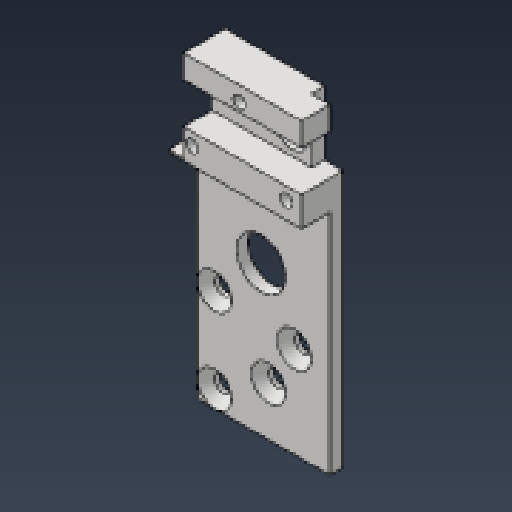
# Autodesk Inventor part: RightGearboxCover
Saved by Autodesk Inventor 2026.2 (Build 302298010, 298A)
## iProperties
Created: 2026-04-04
Part Number: RightGearboxCover
Material: Generic
Document SubType Name: Modeling
Designer: szymo
Density: 1 g/cm^3
Appearance: Default
Author: szymo
Autodesk Inventor part; units mm, degrees
ref_plane "YZ Plane" through (0, 0, 0) normal (1, 0, 0) x (0, 1, 0)
ref_plane "XZ Plane" through (0, 0, 0) normal (0, 1, 0) x (-1, 0, 0)
ref_plane "XY Plane" through (0, 0, 0) normal (0, 0, 1) x (1, 0, 0)
ref_plane "Work Plane1" through (0, -65.2958, -0.3) normal (0, 0, 1) x (1, 0, 0)
sketch "Sketch1" plane through (0, 0, 0) normal (0, 0, 1) x (1, 0, 0)
  circle A0 centre (13, -35.0012) radius 5
  circle A1 centre (13, -35.0012) radius 5.6
  circle A2 centre (8.3716, -9.3577) radius 1.0564
  circle A3 centre (20.6284, -19.6423) radius 1.0564 construction
  circle A4 centre (14.5, -14.5) radius 5 construction
  circle A5 centre (14.5, -14.5) radius 13.85 construction
  circle A6 centre (14.5, -14.5) radius 14.5 construction
  circle A7 centre (14.5, -55.2958) radius 14.5 construction
  circle A8 centre (14.5, -55.2958) radius 13.85 construction
  line L0 (27, 0) -> (0, 0)
  line L1 (0, 0) -> (0, -65.2958)
  line L2 (0, -65.2958) -> (27, -65.2958)
  line L3 (27, -65.2958) -> (27, 0)
  line L4 (1, -17) -> (1, -13.9)
  line L5 (1, -13.9) -> (0, -13.9)
  line L6 (0, -13.9) -> (0, -18)
  line L7 (0, -18) -> (2.4477, -18)
  arc A9 (2.5, -17.9298) -> (2.4477, -18) centre (9.2084, -22.9852) ccw
  line L8 (2.5, -17.9298) -> (2.5, -17)
  line L9 (2.5, -17) -> (1, -17)
  line L10 (3, 0) -> (3, -18.5)
  line L11 (3, -18.5) -> (0, -18.5)
  line L12 (3, -3) -> (27, -3)
  line L13 (27, -13) -> (3, -13)
  line L14 (23.2, 0) -> (23.2, -39.2749)
  arc A10 (9.6825, -42.5548) -> (9.605, -43.9808) centre (15.5954, -43.5915) ccw
  arc A11 (9.605, -43.9808) -> (10.0796, -44.1462) centre (13, -35.0012) ccw
  arc A12 (10.0796, -44.1462) -> (10.905, -42.9808) centre (5.6283, -40.1185) ccw
  arc A13 (10.905, -42.9808) -> (11.3255, -43.0795) centre (13, -35.0012) ccw
  arc A14 (11.3255, -43.0795) -> (11.5461, -44.4905) centre (17.3247, -42.8642) ccw
  arc A15 (11.5461, -44.4905) -> (12.0447, -44.5536) centre (13, -35.0012) ccw
  arc A16 (12.0447, -44.5536) -> (12.6098, -43.242) centre (6.8533, -41.5393) ccw
  arc A17 (12.6098, -43.242) -> (13.0416, -43.2511) centre (13, -35.0012) ccw
  arc A18 (13.0416, -43.2511) -> (13.5508, -44.5854) centre (18.865, -41.7932) ccw
  arc A19 (13.5508, -44.5854) -> (14.0517, -44.5434) centre (13, -35.0012) ccw
  arc A20 (14.0517, -44.5434) -> (14.3317, -43.143) centre (8.347, -42.6744) ccw
  arc A21 (14.3317, -43.143) -> (14.756, -43.0622) centre (13, -35.0012) ccw
  arc A22 (14.756, -43.0622) -> (15.5314, -44.2614) centre (20.1489, -40.4254) ccw
  arc A23 (15.5314, -44.2614) -> (16.0126, -44.1162) centre (13, -35.0012) ccw
  arc A24 (16.0126, -44.1162) -> (15.9954, -42.6882) centre (10.044, -43.4742) ccw
  arc A25 (15.9954, -42.6882) -> (16.3936, -42.5209) centre (13, -35.0012) ccw
  arc A26 (16.3936, -42.5209) -> (17.4014, -43.5327) centre (21.1205, -38.8205) ccw
  arc A27 (17.4014, -43.5327) -> (17.8419, -43.2907) centre (13, -35.0012) ccw
  arc A28 (17.8419, -43.2907) -> (17.5281, -41.8975) centre (11.8702, -43.9036) ccw
  arc A29 (17.5281, -41.8975) -> (17.8829, -41.651) centre (13, -35.0012) ccw
  arc A30 (17.8829, -41.651) -> (19.0791, -42.4312) centre (21.7371, -37.0487) ccw
  arc A31 (19.0791, -42.4312) -> (19.4596, -42.1029) centre (13, -35.0012) ccw
  arc A32 (19.4596, -42.1029) -> (18.863, -40.8053) centre (13.7458, -43.944) ccw
  arc A33 (18.863, -40.8053) -> (19.1587, -40.4905) centre (13, -35.0012) ccw
  arc A34 (19.1587, -40.4905) -> (20.491, -41.0049) centre (21.9719, -35.1874) ccw
  arc A35 (20.491, -41.0049) -> (20.795, -40.6047) centre (13, -35.0012) ccw
  arc A36 (20.795, -40.6047) -> (19.9416, -39.4595) centre (15.5888, -43.5935) ccw
  arc A37 (19.9416, -39.4595) -> (20.1654, -39.0901) centre (13, -35.0012) ccw
  arc A38 (20.1654, -39.0901) -> (21.5756, -39.3163) centre (21.8145, -33.318) ccw
  arc A39 (21.5756, -39.3163) -> (21.7896, -38.8615) centre (13, -35.0012) ccw
  arc A40 (21.7896, -38.8615) -> (20.7169, -37.9188) centre (17.3187, -42.8675) ccw
  arc A41 (20.7169, -37.9188) -> (20.859, -37.5109) centre (13, -35.0012) ccw
  arc A42 (20.859, -37.5109) -> (22.2853, -37.439) centre (21.272, -31.5221) ccw
  arc A43 (22.2853, -37.439) -> (22.4002, -36.9497) centre (13, -35.0012) ccw
  arc A44 (22.4002, -36.9497) -> (21.1548, -36.2506) centre (18.8598, -41.7976) ccw
  arc A45 (21.1548, -36.2506) -> (21.2091, -35.8221) centre (13, -35.0012) ccw
  arc A46 (21.2091, -35.8221) -> (22.5893, -35.4552) centre (20.3678, -29.8783) ccw
  arc A47 (22.5893, -35.4552) -> (22.5999, -34.9527) centre (13, -35.0012) ccw
  arc A48 (22.5999, -34.9527) -> (21.2364, -34.5278) centre (20.1448, -40.4308) ccw
  arc A49 (21.2364, -34.5278) -> (21.2003, -34.0974) centre (13, -35.0012) ccw
  arc A50 (21.2003, -34.0974) -> (22.4741, -33.4516) centre (19.1417, -28.4584) ccw
  arc A51 (22.4741, -33.4516) -> (22.38, -32.9579) centre (13, -35.0012) ccw
  arc A52 (22.38, -32.9579) -> (20.958, -32.8257) centre (21.1176, -38.8267) ccw
  arc A53 (20.958, -32.8257) -> (20.8332, -32.4122) centre (13, -35.0012) ccw
  arc A54 (20.8332, -32.4122) -> (21.9449, -31.5157) centre (17.6472, -27.3244) ccw
  arc A55 (21.9449, -31.5157) -> (21.7502, -31.0523) centre (13, -35.0012) ccw
  arc A56 (21.7502, -31.0523) -> (20.3318, -31.2187) centre (21.7355, -37.0553) ccw
  arc A57 (20.3318, -31.2187) -> (20.1238, -30.8402) centre (13, -35.0012) ccw
  arc A58 (20.1238, -30.8402) -> (21.0247, -29.7321) centre (15.9496, -26.526) ccw
  arc A59 (21.0247, -29.7321) -> (20.738, -29.3193) centre (13, -35.0012) ccw
  arc A60 (20.738, -29.3193) -> (19.3852, -29.777) centre (21.9717, -35.1942) ccw
  arc A61 (19.3852, -29.777) -> (19.103, -29.45) centre (13, -35.0012) ccw
  arc A62 (19.103, -29.45) -> (19.7539, -28.1788) centre (14.123, -26.0979) ccw
  arc A63 (19.7539, -28.1788) -> (19.3876, -27.8347) centre (13, -35.0012) ccw
  arc A64 (19.3876, -27.8347) -> (18.1595, -28.5636) centre (21.8158, -33.3247) ccw
  arc A65 (18.1595, -28.5636) -> (17.8155, -28.3024) centre (13, -35.0012) ccw
  arc A66 (17.8155, -28.3024) -> (18.1878, -26.9237) centre (12.2474, -26.059) ccw
  arc A67 (18.1878, -26.9237) -> (17.758, -26.6632) centre (13, -35.0012) ccw
  arc A68 (17.758, -26.6632) -> (16.7083, -27.6316) centre (21.2746, -31.5284) ccw
  arc A69 (16.7083, -27.6316) -> (16.3175, -27.4476) centre (13, -35.0012) ccw
  arc A70 (16.3175, -27.4476) -> (16.395, -26.0216) centre (10.4046, -26.4109) ccw
  arc A71 (16.395, -26.0216) -> (15.9204, -25.8562) centre (13, -35.0012) ccw
  arc A72 (15.9204, -25.8562) -> (15.095, -27.0216) centre (20.3717, -29.8839) ccw
  arc A73 (15.095, -27.0216) -> (14.6745, -26.9229) centre (13, -35.0012) ccw
  arc A74 (14.6745, -26.9229) -> (14.4539, -25.5119) centre (8.6753, -27.1382) ccw
  arc A75 (14.4539, -25.5119) -> (13.9553, -25.4488) centre (13, -35.0012) ccw
  arc A76 (13.9553, -25.4488) -> (13.3902, -26.7604) centre (19.1467, -28.4631) ccw
  arc A77 (13.3902, -26.7604) -> (12.9584, -26.7513) centre (13, -35.0012) ccw
  arc A78 (12.9584, -26.7513) -> (12.4492, -25.417) centre (7.135, -28.2092) ccw
  arc A79 (12.4492, -25.417) -> (11.9483, -25.459) centre (13, -35.0012) ccw
  arc A80 (11.9483, -25.459) -> (11.6683, -26.8594) centre (17.653, -27.328) ccw
  arc A81 (11.6683, -26.8594) -> (11.244, -26.9402) centre (13, -35.0012) ccw
  arc A82 (11.244, -26.9402) -> (10.4686, -25.741) centre (5.8511, -29.577) ccw
  arc A83 (10.4686, -25.741) -> (9.9874, -25.8861) centre (13, -35.0012) ccw
  arc A84 (9.9874, -25.8861) -> (10.0046, -27.3142) centre (15.956, -26.5282) ccw
  arc A85 (10.0046, -27.3142) -> (9.6064, -27.4815) centre (13, -35.0012) ccw
  arc A86 (9.6064, -27.4815) -> (8.5986, -26.4696) centre (4.8795, -31.1819) ccw
  arc A87 (8.5986, -26.4696) -> (8.1581, -26.7117) centre (13, -35.0012) ccw
  arc A88 (8.1581, -26.7117) -> (8.4719, -28.1049) centre (14.1298, -26.0988) ccw
  arc A89 (8.4719, -28.1049) -> (8.1171, -28.3514) centre (13, -35.0012) ccw
  arc A90 (8.1171, -28.3514) -> (6.9209, -27.5712) centre (4.2629, -32.9537) ccw
  arc A91 (6.9209, -27.5712) -> (6.5404, -27.8995) centre (13, -35.0012) ccw
  arc A92 (6.5404, -27.8995) -> (7.137, -29.1971) centre (12.2542, -26.0584) ccw
  arc A93 (7.137, -29.1971) -> (6.8413, -29.5119) centre (13, -35.0012) ccw
  arc A94 (6.8413, -29.5119) -> (5.509, -28.9975) centre (4.0281, -34.815) ccw
  arc A95 (5.509, -28.9975) -> (5.205, -29.3977) centre (13, -35.0012) ccw
  arc A96 (5.205, -29.3977) -> (6.0584, -30.5429) centre (10.4112, -26.4089) ccw
  arc A97 (6.0584, -30.5429) -> (5.8346, -30.9123) centre (13, -35.0012) ccw
  arc A98 (5.8346, -30.9123) -> (4.4244, -30.6861) centre (4.1855, -36.6844) ccw
  arc A99 (4.4244, -30.6861) -> (4.2104, -31.1409) centre (13, -35.0012) ccw
  arc A100 (4.2104, -31.1409) -> (5.2831, -32.0836) centre (8.6813, -27.1349) ccw
  arc A101 (5.2831, -32.0836) -> (5.141, -32.4915) centre (13, -35.0012) ccw
  arc A102 (5.141, -32.4915) -> (3.7147, -32.5634) centre (4.728, -38.4803) ccw
  arc A103 (3.7147, -32.5634) -> (3.5998, -33.0527) centre (13, -35.0012) ccw
  arc A104 (3.5998, -33.0527) -> (4.8452, -33.7518) centre (7.1402, -28.2047) ccw
  arc A105 (4.8452, -33.7518) -> (4.7909, -34.1803) centre (13, -35.0012) ccw
  arc A106 (4.7909, -34.1803) -> (3.4107, -34.5472) centre (5.6322, -40.1241) ccw
  arc A107 (3.4107, -34.5472) -> (3.4001, -35.0497) centre (13, -35.0012) ccw
  arc A108 (3.4001, -35.0497) -> (4.7636, -35.4746) centre (5.8552, -29.5716) ccw
  arc A109 (4.7636, -35.4746) -> (4.7997, -35.905) centre (13, -35.0012) ccw
  arc A110 (4.7997, -35.905) -> (3.5259, -36.5508) centre (6.8583, -41.544) ccw
  arc A111 (3.5259, -36.5508) -> (3.62, -37.0445) centre (13, -35.0012) ccw
  arc A112 (3.62, -37.0445) -> (5.042, -37.1767) centre (4.8824, -31.1757) ccw
  arc A113 (5.042, -37.1767) -> (5.1668, -37.5902) centre (13, -35.0012) ccw
  arc A114 (5.1668, -37.5902) -> (4.0551, -38.4867) centre (8.3528, -42.678) ccw
  arc A115 (4.0551, -38.4867) -> (4.2498, -38.9501) centre (13, -35.0012) ccw
  arc A116 (4.2498, -38.9501) -> (5.6682, -38.7837) centre (4.2645, -32.9471) ccw
  arc A117 (5.6682, -38.7837) -> (5.8762, -39.1622) centre (13, -35.0012) ccw
  arc A118 (5.8762, -39.1622) -> (4.9753, -40.2703) centre (10.0504, -43.4764) ccw
  arc A119 (4.9753, -40.2703) -> (5.262, -40.6831) centre (13, -35.0012) ccw
  arc A120 (5.262, -40.6831) -> (6.6148, -40.2254) centre (4.0283, -34.8082) ccw
  arc A121 (6.6148, -40.2254) -> (6.897, -40.5524) centre (13, -35.0012) ccw
  arc A122 (6.897, -40.5524) -> (6.2461, -41.8236) centre (11.877, -43.9045) ccw
  arc A123 (6.2461, -41.8236) -> (6.6124, -42.1677) centre (13, -35.0012) ccw
  arc A124 (6.6124, -42.1677) -> (7.8405, -41.4388) centre (4.1842, -36.6777) ccw
  arc A125 (7.8405, -41.4388) -> (8.1845, -41.7) centre (13, -35.0012) ccw
  arc A126 (8.1845, -41.7) -> (7.8122, -43.0787) centre (13.7526, -43.9434) ccw
  arc A127 (7.8122, -43.0787) -> (8.242, -43.3392) centre (13, -35.0012) ccw
  arc A128 (8.242, -43.3392) -> (9.2917, -42.3708) centre (4.7254, -38.474) ccw
  arc A129 (9.2917, -42.3708) -> (9.6825, -42.5548) centre (13, -35.0012) ccw
  circle A130 centre (13, -35.0012) radius 9.6 construction
  point P0 (0, 0)
  point P1 (23.2, -13)
  point P2 (23.2, -3)
extrude "Extrusion1" add sketch "Sketch1" against normal up to surface (0.3 mm away) contours A2 | L14 L12 L10 L0 | L14 L13 L10 L12 | L3 L2 L1 L11 L10 L13 | A129 A128 A127 A126 A125 A124 A123 A122 A121 A120 A119 A118 A117 A116 A115 A114 A113 A112 A111 A110 A109 A108 A107 A106 A105 A104 A103 A102 A101 A100 A99 A98 A97 A96 A95 A94 A93 A92 A91 A90 A89 A88 A87 A86 A85 A84 A83 A82 A81 A80 A79 A78 A77 A76 A75 A74 A73 A72 A71 A70 A69 A68 A67 A66 A65 A64 A63 A62 A61 A60 A59 A58 A57 A56 A55 A54 A53 A52 A51 A50 A49 A48 A47 A46 A45 A44 A43 A42 A41 A40 A39 A38 A37 A36 A35 A34 A33 A32 A31 A30 A29 A28 A27 A26 A25 A24 A23 A22 A21 A20 A19 A18 A17 A16 A15 A14 A13 A12 A11 A10
ref_plane "Work Plane2" through (8.0794, -39.9218, 2.4) normal (0, 0, 1) x (0.9996763, -0.0254413, 0)
extrude "Extrusion2" add sketch "Sketch1" along normal up to surface (2.4 mm away) contours A1 | A2 | L14 L12 L10 L0 | L14 L13 L10 L12 | L3 L2 L1 L11 L10 L13 | A129 A128 A127 A126 A125 A124 A123 A122 A121 A120 A119 A118 A117 A116 A115 A114 A113 A112 A111 A110 A109 A108 A107 A106 A105 A104 A103 A102 A101 A100 A99 A98 A97 A96 A95 A94 A93 A92 A91 A90 A89 A88 A87 A86 A85 A84 A83 A82 A81 A80 A79 A78 A77 A76 A75 A74 A73 A72 A71 A70 A69 A68 A67 A66 A65 A64 A63 A62 A61 A60 A59 A58 A57 A56 A55 A54 A53 A52 A51 A50 A49 A48 A47 A46 A45 A44 A43 A42 A41 A40 A39 A38 A37 A36 A35 A34 A33 A32 A31 A30 A29 A28 A27 A26 A25 A24 A23 A22 A21 A20 A19 A18 A17 A16 A15 A14 A13 A12 A11 A10
sketch "Sketch2" plane through (27, -65.2958, -0.3) normal (0, 0, -1) x (-1, 0, 0)
  circle A0 centre (12.5, 50.7958) radius 1.15 projected
  circle A1 centre (12.5, 50.7958) radius 1.65
  circle A2 centre (17.7916, 42.3106) radius 3 projected
  point P0 (27, 65.2958)
  dimension "d9" = 0.5
  constraints: 1 centre point
  measures "d9" radial gap between concentric circles of A0 A1
extrude "Extrusion3" cut sketch "Sketch2" against normal blind 2 contours A0 | A1
ref_plane "Work Plane3" through (1, -19, 8.2) normal (0, 0, -1) x (0, 1, 0)
sketch "Sketch4" plane through (0, -65.2958, 2.4) normal (0, 0, 1) x (1, 0, 0)
  circle A0 centre (14.325, 62.2958) radius 0.75 projected
  circle A1 centre (4.725, 49.7467) radius 0.75 projected
  circle A2 centre (23.925, 49.7467) radius 0.75 projected
  line L0 (23.7668, 46.2958) -> (4.8832, 46.2958) projected
  arc A3 (4.8832, 46.2958) -> (4.8444, 46.2989) centre (4.825, 45.7992) ccw projected
  arc A4 (1, 50.2958) -> (4.8444, 46.2989) centre (5, 50.2958) ccw projected
  line L1 (1, 60.2958) -> (1, 50.2958) projected
  arc A5 (6, 65.2958) -> (1, 60.2958) centre (6, 60.2958) ccw projected
  line L2 (22.65, 65.2958) -> (6, 65.2958) projected
  arc A6 (27.65, 60.2958) -> (22.65, 65.2958) centre (22.65, 60.2958) ccw projected
  line L3 (27.65, 50.2958) -> (27.65, 60.2958) projected
  arc A7 (23.8056, 46.2989) -> (27.65, 50.2958) centre (23.65, 50.2958) ccw projected
  arc A8 (23.8056, 46.2989) -> (23.7668, 46.2958) centre (23.825, 45.7992) ccw projected
  line L4 (23.2, 65.2958) -> (23.2, 52.2958) projected
  line L5 (23.2, 52.2958) -> (3, 52.2958)
  line L6 (3, 46.7958) -> (3, 65.2958) projected
  line L7 (27, 52.2958) -> (27, 0) projected
  line L8 (27, 46.2958) -> (0, 46.2958)
  line L9 (0, 0) -> (0, 46.7958) projected
  line L10 (23.2, 60.5458) -> (3, 60.5458)
  line L11 (3, 65.2958) -> (23.2, 65.2958) projected
  line L12 (3, 65.2958) -> (23.2, 65.2958) projected
  line L13 (0, 46.7958) -> (3, 46.7958) projected
  line L14 (0, 46.7958) -> (3, 46.7958) projected
  line L15 (27, 52.2958) -> (27, 0) projected
  line L16 (27, 52.2958) -> (27, 0) projected
  line L17 (27, 62.2958) -> (23.8, 62.2958) projected
  line L18 (27, 62.2958) -> (23.8, 62.2958) projected
  line L19 (23.2, 52.2958) -> (27, 52.2958) projected
  line L20 (23.2, 52.2958) -> (27, 52.2958) projected
  line L21 (23.8, 62.2958) -> (23.8, 65.2958)
  point P0 (0, 65.2958)
  point P1 (27, 52.2958)
  point P2 (0, 46.7958)
  point P3 (4.8832, 46.2958)
  point P4 (27, 65.2958)
  point P5 (22.65, 65.2958)
  point P6 (23.8, 62.2958)
  point P7 (27, 62.2958)
  point P8 (23.8, 62.2958)
  point P9 (23.2, 65.2958)
  dimension "d15" = 1
  constraints: 6 end point, 5 point on line, 1 collinear, 1 horizontal, 1 parallel, 1 perpendicular, 5 other
  measures "d15" distance edge to line of A0 L10
extrude "Extrusion4" add sketch "Sketch4" along normal up to surface (5.8 mm away) contours A0 | A1 | A2 | L0 A3 A4 L6 L5 L19 L7 A7 A8 | A8 A7 L7 L8 | L8 L9 L13 L6 A4 A3 | L6 A5 L2 A6 L4 L10 | L6 L11 A5 | A6 L11 L4
sketch "Sketch5" plane through (27, -65.2958, -0.3) normal (0, 0, -1) x (-1, 0, 0)
  circle A0 centre (12.675, 62.2958) radius 0.75 projected
  circle A1 centre (22.275, 49.7467) radius 0.75 projected
  circle A2 centre (3.075, 49.7467) radius 0.75 projected
  line L0 (3.2332, 46.2958) -> (22.1168, 46.2958) projected
  arc A3 (22.1556, 46.2989) -> (22.1168, 46.2958) centre (22.175, 45.7992) ccw projected
  arc A4 (22.1556, 46.2989) -> (26, 50.2958) centre (22, 50.2958) ccw projected
  line L1 (26, 60.2958) -> (26, 50.2958) projected
  arc A5 (26, 60.2958) -> (21, 65.2958) centre (21, 60.2958) ccw projected
  line L2 (4.35, 65.2958) -> (21, 65.2958) projected
  arc A6 (4.35, 65.2958) -> (-0.65, 60.2958) centre (4.35, 60.2958) ccw projected
  line L3 (-0.65, 50.2958) -> (-0.65, 60.2958) projected
  arc A7 (-0.65, 50.2958) -> (3.1944, 46.2989) centre (3.35, 50.2958) ccw projected
  arc A8 (3.2332, 46.2958) -> (3.1944, 46.2989) centre (3.175, 45.7992) ccw projected
  point P0 (27, 65.2958)
hole "Hole1" at (23.925, -15.5491, -0.3) at (14.325, -3, -0.3) at (4.725, -15.5491, -0.3) direction (0, 0, 1) diameter 3 depth 4.5 counterbore diameter 3.5 counterbore depth 0.5
hole "Hole2" at (23.925, -15.5491, -0.3) at (14.325, -3, -0.3) at (4.725, -15.5491, -0.3) direction (0, 0, 1) diameter 2.5 end through all
hole "Hole3" at (9.2084, -22.9852, -0.3) direction (0, 0, 1) diameter 2.5 depth 2.5
sketch "Sketch6" plane through (0, -65.2958, 2.4) normal (0, 0, 1) x (1, 0, 0)
  circle A0 centre (19.7, 18.5746) radius 2.25 projected
  circle A1 centre (14.5, 10) radius 2.25 projected
  circle A2 centre (3.5, 20.703) radius 2.25 projected
  circle A3 centre (3.5, 20.703) radius 2 projected
  circle A4 centre (3.5, 3.5) radius 2 projected
  circle A5 centre (19.2, 57.0458) radius 2 projected
  point P0 (0, 65.2958)
  point P1 (19.7, 61.7958)
hole "Hole4" at (19.7, -46.7213, 2.4) at (14.5, -55.2958, 2.4) at (3.5, -61.7958, 2.4) at (3.5, -44.5929, 2.4) at (19.2, -8.25, 2.4) direction (0, 0, -1) diameter 3.4 depth 7 countersink diameter 7 countersink angle 90 clearance for "Countersunk Flat Head Screw ISO 2009/7046" size "M3" standard "ISO"
sketch "Sketch7" plane through (3, 0, -0.3) normal (0, 1, 0) x (1, 0, 0)
  line L0 (20.2, 0) -> (24, 0) projected
  line L1 (20.2, 0) -> (20.2, -2.7) projected
  line L2 (0, -2.7) -> (20.2, -2.7) projected
  line L3 (0, -2.7) -> (0, -8.5) projected
  line L4 (24, -8.5) -> (0, -8.5) projected
  line L5 (24, 0) -> (24, -8.5) projected
  line L6 (20.2, 9) -> (20.2, -2.6) projected
  line L7 (20.2, -2.6) -> (21, -2.6) projected
  line L8 (21, 9) -> (21, -2.6) projected
  line L9 (20.2, 9) -> (21, 9) projected
  line L10 (24, 0) -> (24, -8.5) projected
  line L11 (20.2, -8.5) -> (24, -8.5)
  line L12 (24, -8.5) -> (24, -2.7)
  line L13 (24, -2.7) -> (20.2, -2.7)
  line L14 (20.2, -2.7) -> (20.2, -8.5)
  point P0 (-3, -0.3)
  point P1 (24, -2.7)
  dimension "d47" = 0.1
  dimension "d48" = 0
  constraints: 8 end point, 2 parallel, 2 point on line, 1 horizontal, 1 perpendicular
  measures "d47" distance between parallel lines of L7 L13
  measures "d48" distance between parallel lines of L1 L14
extrude "Extrusion5" add sketch "Sketch7" against normal up to surface (4.75 mm away) contours L13 L5 L4 L14
body "Solid1"
